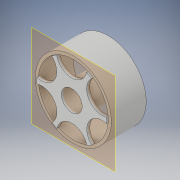
# Autodesk Inventor part: Wheel
Saved by Autodesk Inventor 2017 (Build 210142000, 142)
## iProperties
Created: 2020-02-18
Part Number: Wheel
Material: Generic
Document SubType Name: Modeling
Designer: 10042265
Density: 1 g/cm^3
Appearance: Default
Author: 10042265
Autodesk Inventor part; units mm, degrees
ref_plane "YZ Plane" through (0, 0, 0) normal (1, 0, 0) x (0, 1, 0)
ref_plane "XZ Plane" through (0, 0, 0) normal (0, 1, 0) x (-1, 0, 0)
ref_plane "XY Plane" through (0, 0, 0) normal (0, 0, 1) x (1, 0, 0)
sketch "Sketch1" plane through (0, 0, 0) normal (0, 0, 1) x (1, 0, 0)
  circle A0 centre (0, 0) radius 5.588
  circle A1 centre (0, 0) radius 4.318
  circle A2 centre (0, 0) radius 14.478
  circle A3 centre (0, 0) radius 15.748
  dimension "d0" = 11.176
  dimension "d1" = 1.27
  dimension "d2" = 8.89
  dimension "d3" = 1.27
  constraints: 4 centre point, 1 coincident
  measures "d0" diameter of A0
  measures "d1" radial gap between concentric circles of A0 A1
  measures "d2" radial gap between concentric circles of A0 A2
  measures "d3" radial gap between concentric circles of A2 A3
extrude "Extrusion1" add sketch "Sketch1" along normal blind 14.478
ref_plane "Work Plane1" through (0, 0, 14.478) normal (0, 0, 1) x (1, 0, 0)
sketch "Sketch2" plane through (0, 0, 14.478) normal (0, 0, 1) x (1, 0, 0)
  circle A0 centre (0, 0) radius 14.478 projected
  circle A1 centre (0, 0) radius 15.748 projected
  circle A2 centre (0, 0) radius 4.318 projected
  circle A3 centre (0, 0) radius 5.588 projected
extrude "Extrusion2" add sketch "Sketch2" along normal mid plane 1.27 contours A0 | A3
sketch "Sketch3" plane through (0, 0, 15.113) normal (0, 0, 1) x (1, 0, 0)
  circle A0 centre (0, 0) radius 14.478 projected
  circle A1 centre (0, 0) radius 14.478 projected
  arc A2 (-6.2546, 13.0573) -> (6.1362, 13.1134) centre (-0.0655, 14.4779) ccw
  arc A3 (6.1362, 13.1134) -> (-6.2546, 13.0573) centre (0, 0) ccw
  dimension "d9" = 12.7
  constraints: 8 point on circle, 2 centre point, 2 other
  measures "d9" diameter of A2
extrude "Extrusion3" cut sketch "Sketch3" against normal blind 1.27 contours A2 A0 picked at (-1.876, 12.3773)
pattern_circular "Circular Pattern1" count 6 over 360 about axis through (0, 0, 14.478) along (0, 0, 1) of "Extrusion3"
body "Solid1"
